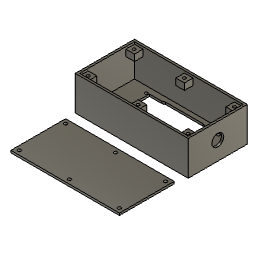
microarcade (Autodesk Fusion 360 design; units mm, degrees)
part number: 2025-05-01-21-42-39-432
Autodesk Fusion 360 part; units mm, degrees
sketch "Sketch1" plane through (0, 0, 0) normal (0, 0, 1) x (1, 0, 0)
  line L0 (33.5, -19.65) -> (-33.5, -19.65) construction
  line L1 (-33.5, -19.65) -> (-33.5, 19.65) construction
  line L2 (-33.5, 19.65) -> (33.5, 19.65) construction
  line L3 (33.5, 19.65) -> (33.5, -19.65) construction
  line L4 (33.5, -19.65) -> (-33.5, 19.65) construction
  line L5 (-33.5, -19.65) -> (33.5, 19.65) construction
  circle A0 centre (-33.5, 19.65) radius 1.375
  circle A1 centre (33.5, 19.65) radius 1.375
  circle A2 centre (-33.5, -19.65) radius 1.375
  circle A3 centre (33.5, -19.65) radius 1.375
  line L6 (31.375, -18.9) -> (-31.375, -18.9) construction
  line L7 (-31.375, -18.9) -> (-31.375, 20.35) construction
  line L8 (-31.375, 20.35) -> (31.375, 20.35) construction
  line L9 (31.375, 20.35) -> (31.375, -18.9)
  line L10 (31.375, -18.9) -> (-31.375, 20.35) construction
  line L11 (-31.375, -18.9) -> (31.375, 20.35) construction
  line L12 (-19.875, 22) -> (-19.875, -25) construction
  line L13 (19.875, 21.8233) -> (19.875, -25.5545) construction
  line L14 (-17.375, 22.5455) -> (-17.375, -22.5266) construction
  line L15 (17.375, 23.3898) -> (17.375, -22.6276) construction
  line L16 (0, 20.35) -> (0, 11.4847) construction
  line L17 (-23.2845, 21.35) -> (29, 21.35) construction
  line L18 (17.375, 21.35) -> (19.875, 20.35)
  line L19 (19.875, 20.35) -> (31.375, 20.35)
  line L20 (31.375, -18.9) -> (-31.375, -18.9)
  line L21 (-31.375, 20.35) -> (-19.875, 20.35)
  line L22 (-19.875, 20.35) -> (-17.375, 21.35)
  line L23 (17.375, 21.35) -> (17.375, 22)
  line L24 (-17.375, 21.35) -> (17.375, 21.35)
  line L25 (31.375, 20.35) -> (31.375, -18.9)
  line L26 (-31.375, 20.35) -> (-31.375, -18.9)
  line L27 (52.5, -27.5) -> (-52.5, -27.5)
  line L28 (-52.5, -27.5) -> (-52.5, 27.5)
  line L29 (-52.5, 27.5) -> (52.5, 27.5)
  line L30 (52.5, 27.5) -> (52.5, -27.5)
  line L31 (52.5, -27.5) -> (-52.5, 27.5) construction
  line L32 (-52.5, -27.5) -> (52.5, 27.5) construction
  circle A4 centre (-42.25, -7.5) radius 3.5
  circle A5 centre (42.25, -7.5) radius 3.5
  line L33 (50.5, 25.5) -> (50.5, -25.5)
  line L34 (50.5, -25.5) -> (-50.5, -25.5)
  line L35 (-50.5, -25.5) -> (-50.5, 25.5)
  line L36 (-50.5, 25.5) -> (50.5, 25.5)
  dimension "d1" = 67
  dimension "d2" = 39.3
  dimension "d3" = 2.75
  dimension "d4" = 2.75
  dimension "d5" = 2.75
  dimension "d6" = 2.75
  dimension "d7" = 62.75
  dimension "d8" = 39.25
  dimension "d9" = 11.5
  dimension "d10" = 11.5
  dimension "d12" = 2.5
  dimension "d13" = 2.5
  dimension "d17" = 0.75
  dimension "d18" = 1
  dimension "d19" = 105
  dimension "d20" = 55
  dimension "d29" = 7
  dimension "d30" = 20
  dimension "d31" = 10.25
  dimension "d32" = 7
  dimension "d33" = 20
  dimension "d34" = 10.25
  dimension "d39" = 2
  constraint horizontal L0
  constraint perpendicular L0 L1
  constraint parallel L0 L2
  constraint parallel L1 L3
  constraint coincident L4 origin
  constraint coincident L5 origin
  constraint coincident L1.end L2.start
  constraint coincident L2.end L3.start
  constraint coincident L0.end L1.start
  constraint coincident L0.start L3.end
  constraint horizontal L6
  constraint perpendicular L6 L7
  constraint parallel L6 L8
  constraint parallel L7 L9
  constraint perpendicular L0 L12
  constraint perpendicular L6 L13
  constraint perpendicular L6 L14
  constraint perpendicular L0 L15
  constraint midpoint L8 L16.start
  constraint perpendicular L2 L16
  constraint coincident origin L16
  constraint parallel L8 L17
  constraint coincident L17 L18.start
  constraint coincident L15 L18.start
  constraint coincident L13 L18.end
  constraint coincident L8 L18.end
  constraint coincident L8 L21.end
  constraint coincident L12 L21.end
  constraint coincident L14 L22.end
  constraint coincident L17 L22.end
  constraint coincident L15 L23.end
  constraint perpendicular L17 L23
  constraint horizontal L27
  constraint perpendicular L27 L28
  constraint parallel L27 L29
  constraint parallel L28 L30
  constraint coincident L31 origin
  constraint coincident L32 origin
  measures "d1" distance of L1.end L2.end
  measures "d2" distance of L0.end L1.end
  measures "d3" diameter of A0
  measures "d4" diameter of A1
  measures "d5" diameter of A2
  measures "d6" diameter of A3
  measures "d7" distance of L7.end L8.end
  measures "d8" distance of L6.end L7.end
  measures "d9" distance of L7 L12
  measures "d10" distance of L9 L13
  measures "d12" distance of L12 L14
  measures "d13" distance of L13 L15
  measures "d17" distance of L0 L6
  measures "d18" distance of L8 L17
  measures "d19" distance of L28.end L29.end
  measures "d20" distance of L27.end L28.end
  measures "d29" diameter of A4
  measures "d30" distance of L27 A4.centre
  measures "d31" distance of L28 A4.centre
  measures "d32" diameter of A5
  measures "d33" distance of L27 A5.centre
  measures "d34" distance of L30 A5.centre
extrude "Extrude1" add sketch "Sketch1" along normal blind 2 contours L27 L28 L29 L30 | A4 | A5 | L33 L34 L35 L36 makes body 1
sketch "Sketch2" plane through (0, 0, 2) normal (0, 0, 1) x (-1, 0, 0)
  circle A0 centre (33.5, 19.65) radius 1.375
  circle A1 centre (33.5, -19.65) radius 1.375
  circle A2 centre (-33.5, -19.65) radius 1.375
  circle A3 centre (-33.5, 19.65) radius 1.375
  line L0 (31.375, -20.35) -> (19.875, -20.35)
  line L1 (19.875, -20.35) -> (17.375, -21.35)
  line L2 (17.375, -21.35) -> (-17.375, -21.35)
  line L3 (-17.375, -21.35) -> (-19.875, -20.35)
  line L4 (-19.875, -20.35) -> (-31.375, -20.35)
  line L5 (-31.375, -20.35) -> (-31.375, 18.9)
  line L6 (-31.375, 18.9) -> (31.375, 18.9)
  line L7 (31.375, 18.9) -> (31.375, -20.35)
  line L8 (-52.5, -27.5) -> (52.5, -27.5)
  line L9 (52.5, -27.5) -> (52.5, 27.5)
  line L10 (52.5, 27.5) -> (-52.5, 27.5)
  line L11 (-52.5, 27.5) -> (-52.5, -27.5)
  line L12 (0, -29) -> (0, 27) construction
  line L13 (22.4113, 21.9) -> (-25, 21.9) construction
  line L14 (9, 7.5969) -> (9, 29.497) construction
  line L15 (-9, 10) -> (-9, 29) construction
  line L16 (11.7573, 19.4) -> (-17.4231, 19.4) construction
  line L17 (9, 19.4) -> (-9, 19.4)
  line L18 (-9, 19.4) -> (-9, 21.9)
  line L19 (-9, 21.9) -> (9, 21.9)
  line L20 (9, 21.9) -> (9, 19.4)
  dimension "d23" = 3
  dimension "d24" = 9
  dimension "d25" = 9
  dimension "d26" = 0.5
  constraint perpendicular L2 L12
  constraint parallel L6 L13
  constraint perpendicular L10 L14
  constraint parallel L12 L15
  constraint horizontal L17
  constraint vertical L18
  constraint horizontal L19
  constraint vertical L20
  constraint coincident L13 L18.end
  constraint coincident L15 L18.end
  constraint coincident L16 L17.start
  constraint coincident L14 L17.start
  measures "d23" distance of L6 L13
  measures "d24" distance of L12 L14
  measures "d25" distance of L12 L15
  measures "d26" distance of L6 L16
extrude "Extrude2" cut sketch "Sketch2" against normal blind 1.75 contours L17 L18 L19 L20 bodies 1
sketch "Sketch3" plane through (0, 0, 0) normal (0, 1, 0) x (1, 0, 0)
extrude "Extrude3" cut sketch "Sketch1" along normal blind 2 contours A5 bodies 1
extrude "Extrude4" cut sketch "Sketch1" along normal blind 2 contours A4 bodies 1
sketch "Sketch4" plane through (0, 0, 0) normal (1, 0, 0) x (0, 1, 0)
sketch "Sketch5" plane through (0, 0, 0) normal (0, 0, 1) x (1, 0, 0)
extrude "Extrude5" add sketch "Sketch1" along normal blind 30 contours L27 L28 L29 L30 bodies 1
sketch "Sketch6" plane through (0, 0, 0) normal (0, 1, 0) x (1, 0, 0)
sketch "Sketch7" plane through (0, 0, 30) normal (0, 0, 1) x (-1, 0, 0)
  line L0 (50.5, 25.5) -> (50.5, -25.5)
  line L1 (50.5, -25.5) -> (-50.5, -25.5)
  line L2 (-50.5, -25.5) -> (-50.5, 25.5)
  line L3 (-50.5, 25.5) -> (50.5, 25.5)
  line L4 (-52.5, -27.5) -> (52.5, -27.5)
  line L5 (52.5, -27.5) -> (52.5, 27.5)
  line L6 (52.5, 27.5) -> (-52.5, 27.5)
  line L7 (-52.5, 27.5) -> (-52.5, -27.5)
  line L8 (-50.5, 25.5) -> (-42.5, 25.5)
  line L9 (-42.5, 25.5) -> (-42.5, 17.5)
  line L10 (-42.5, 17.5) -> (-50.5, 17.5)
  line L11 (-50.5, 17.5) -> (-50.5, 25.5)
  line L12 (50.5, 25.5) -> (42.5, 25.5)
  line L13 (42.5, 25.5) -> (42.5, 17.5)
  line L14 (42.5, 17.5) -> (50.5, 17.5)
  line L15 (50.5, 17.5) -> (50.5, 25.5)
  line L16 (-50.5, -25.5) -> (-42.5, -25.5)
  line L17 (-42.5, -25.5) -> (-42.5, -17.5)
  line L18 (-42.5, -17.5) -> (-50.5, -17.5)
  line L19 (-50.5, -17.5) -> (-50.5, -25.5)
  line L20 (50.5, -25.5) -> (42.5, -25.5)
  line L21 (42.5, -25.5) -> (42.5, -17.5)
  line L22 (42.5, -17.5) -> (50.5, -17.5)
  line L23 (50.5, -17.5) -> (50.5, -25.5)
  line L24 (-4, 25.5) -> (4, 25.5)
  line L25 (4, 25.5) -> (4, 17.5)
  line L26 (4, 17.5) -> (-4, 17.5)
  line L27 (-4, 17.5) -> (-4, 25.5)
  line L28 (0, 40) -> (0, -40) construction
  line L29 (-4, -25.5) -> (4, -25.5)
  line L30 (4, -25.5) -> (4, -17.5)
  line L31 (4, -17.5) -> (-4, -17.5)
  line L32 (-4, -17.5) -> (-4, -25.5)
  line L33 (-46.5, 25.5) -> (-46.5, 17.5) construction
  circle A0 centre (-46.5, 21.5) radius 1.4
  line L34 (0, 25.5) -> (0, 17.5) construction
  circle A1 centre (0, 21.5) radius 1.4
  line L35 (46.5, 25.5) -> (46.5, 17.5) construction
  circle A2 centre (46.5, 21.5) radius 1.4
  line L36 (-46.5, -17.5) -> (-46.5, -25.5) construction
  circle A3 centre (-46.5, -21.5) radius 1.4
  line L37 (0, -17.5) -> (0, -25.5) construction
  circle A4 centre (0, -21.5) radius 1.4
  line L38 (46.5, -17.5) -> (46.5, -25.5) construction
  circle A5 centre (46.5, -21.336) radius 1.4
  dimension "d42" = 8
  dimension "d43" = 8
  dimension "d44" = 8
  dimension "d45" = 8
  dimension "d46" = 8
  dimension "d47" = 8
  dimension "d48" = 8
  dimension "d49" = 8
  dimension "d50" = 8
  dimension "d51" = 8
  dimension "d52" = 4
  dimension "d53" = 8
  dimension "d54" = 8
  dimension "d55" = 4
  dimension "d58" = 2.8
  dimension "d59" = 2.8
  dimension "d60" = 2.8
  dimension "d61" = 2.8
  dimension "d62" = 2.8
  dimension "d63" = 2.8
  constraint horizontal L8
  constraint vertical L9
  constraint horizontal L10
  constraint vertical L11
  constraint coincident L2.end L3.start
  constraint horizontal L12
  constraint vertical L13
  constraint horizontal L14
  constraint vertical L15
  constraint coincident L0.start L3.end
  constraint horizontal L16
  constraint vertical L17
  constraint horizontal L18
  constraint vertical L19
  constraint coincident L1.end L2.start
  constraint horizontal L20
  constraint vertical L21
  constraint horizontal L22
  constraint vertical L23
  constraint coincident L0.end L1.start
  constraint horizontal L24
  constraint vertical L25
  constraint horizontal L26
  constraint vertical L27
  constraint coincident L3 L24.start
  constraint perpendicular L4 L28
  constraint horizontal L29
  constraint vertical L30
  constraint horizontal L31
  constraint vertical L32
  constraint coincident L1 L29.start
  constraint midpoint L8 L33.start
  constraint midpoint L10 L33.end
  constraint midpoint L33 A0.centre
  constraint midpoint L24 L34.start
  constraint midpoint L26 L34.end
  constraint midpoint L34 A1.centre
  constraint midpoint L12 L35.start
  constraint midpoint L14 L35.end
  constraint midpoint L35 A2.centre
  constraint midpoint L18 L36.start
  constraint midpoint L16 L36.end
  constraint midpoint L36 A3.centre
  constraint midpoint L31 L37.start
  constraint midpoint L29 L37.end
  constraint midpoint L37 A4.centre
  constraint midpoint L22 L38.start
  constraint midpoint L20 L38.end
  constraint coincident L38 A5.centre
  measures "d42" distance of L2.end L8.end
  measures "d43" distance of L2.end L10.end
  measures "d44" distance of L0.start L12.end
  measures "d45" distance of L12 L14
  measures "d46" distance of L1.end L16.end
  measures "d47" distance of L1.end L18.end
  measures "d48" distance of L20 L22
  measures "d49" distance of L21 L23
  measures "d50" distance of L24.start L26.end
  measures "d51" distance of L25.end L26.end
  measures "d52" distance of L25 L28
  measures "d53" distance of L29.start L31.end
  measures "d54" distance of L29.start L29.end
  measures "d55" distance of L28 L30
  measures "d58" diameter of A0
  measures "d59" diameter of A1
  measures "d60" diameter of A2
  measures "d61" diameter of A3
  measures "d62" diameter of A4
  measures "d63" diameter of A5
extrude "Extrude6" add sketch "Sketch7" against normal blind 6 contours L0 L3 L12 L13 L14 L15 | L0 L1 L20 L21 L22 L23 | L3 L24 L25 L26 L27 | L2 L3 L8 L9 L10 L11 | L1 L29 L30 L31 L32 | L1 L2 L16 L17 L18 L19 | A0 | A1 | A2 | A3 | A4 | A5 bodies 1
extrude "Extrude7" cut sketch "Sketch7" against normal blind 7 contours A0 | A1 | A2 | A3 | A4 | A5 bodies 1
sketch "Sketch8" plane through (52.5, 0, 0) normal (1, 0, 0) x (0, 1, 0)
  line L0 (-27.5, 0) -> (27.5, 0)
  line L1 (27.5, 0) -> (27.5, 30)
  line L2 (27.5, 30) -> (-27.5, 30)
  line L3 (-27.5, 30) -> (-27.5, 0)
  line L4 (0, 30) -> (0, 0) construction
  circle A0 centre (0, 17) radius 5.5
  dimension "d66" = 11
  dimension "d95" = 13
  constraint midpoint L2 L4.start
  constraint coincident L4.end origin
  measures "d66" diameter of A0
  measures "d95" distance of L4.start A0.centre
extrude "Extrude8" cut sketch "Sketch8" against normal blind 2 contours A0 bodies 1
sketch "Sketch9" plane through (0, 0, 0) normal (0, 0, 1) x (1, 0, 0)
sketch "Sketch11" plane through (0, 0, 0) normal (0, 0, 1) x (1, 0, 0)
  line L0 (-50.5, -38.5133) -> (50.5, -38.5133)
  line L1 (50.5, -38.5133) -> (50.5, -89.5133)
  line L2 (50.5, -89.5133) -> (-50.5, -89.5133)
  line L3 (-50.5, -89.5133) -> (-50.5, -38.5133)
  line L4 (-50.5, -38.5133) -> (-46.5, -38.5133)
  line L5 (-46.5, -38.5133) -> (-46.5, -42.5133) construction
  line L6 (-46.5, -42.5133) -> (-50.5, -42.5133) construction
  line L7 (-50.5, -42.5133) -> (-50.5, -38.5133)
  line L8 (-50.5, -38.5133) -> (0, -38.5133)
  line L9 (0, -89.5133) -> (0, -38.5133) construction
  line L10 (-2, -38.5133) -> (-2, -89.5133) construction
  line L11 (-2, -38.5133) -> (2, -38.5133)
  line L12 (2, -38.5133) -> (2, -42.5133) construction
  line L13 (2, -42.5133) -> (-2, -42.5133) construction
  line L14 (-2, -42.5133) -> (-2, -38.5133) construction
  line L15 (-52.5, 27.5) -> (-52.5, -27.5)
  line L16 (50.5, -38.5133) -> (46.5, -38.5133)
  line L17 (46.5, -38.5133) -> (46.5, -42.5133) construction
  line L18 (46.5, -42.5133) -> (50.5, -42.5133) construction
  line L19 (50.5, -42.5133) -> (50.5, -38.5133)
  line L20 (-50.5, -89.5133) -> (-46.5, -89.5133)
  line L21 (-46.5, -89.5133) -> (-46.5, -85.5133) construction
  line L22 (-46.5, -85.5133) -> (-50.5, -85.5133) construction
  line L23 (-50.5, -85.5133) -> (-50.5, -89.5133)
  line L24 (-2, -89.5133) -> (2, -89.5133)
  line L25 (2, -89.5133) -> (2, -85.5133) construction
  line L26 (2, -85.5133) -> (-2, -85.5133) construction
  line L27 (-2, -85.5133) -> (-2, -89.5133)
  line L28 (50.5, -89.5133) -> (46.5, -89.5133)
  line L29 (46.5, -89.5133) -> (46.5, -85.5133) construction
  line L30 (46.5, -85.5133) -> (50.5, -85.5133) construction
  line L31 (50.5, -85.5133) -> (50.5, -89.5133)
  circle A0 centre (-46.5, -42.5133) radius 1.5
  circle A1 centre (0, -42.5133) radius 1.5
  circle A2 centre (46.5, -42.5133) radius 1.5
  circle A3 centre (-46.5, -85.5133) radius 1.5
  circle A4 centre (0, -85.5133) radius 1.5
  circle A5 centre (46.5, -85.5133) radius 1.5
  line L32 (-50.5, -17.5) -> (-50.5, -25.5)
  dimension "d69" = 51
  dimension "d70" = 101
  dimension "d72" = 4
  dimension "d73" = 4
  dimension "d74" = 2
  dimension "d75" = 4
  dimension "d76" = 4
  dimension "d77" = 4
  dimension "d78" = 4
  dimension "d79" = 4
  dimension "d80" = 4
  dimension "d81" = 4
  dimension "d82" = 4
  dimension "d83" = 4
  dimension "d84" = 4
  dimension "d85" = 3
  dimension "d86" = 3
  dimension "d87" = 3
  dimension "d88" = 3
  dimension "d89" = 3
  dimension "d90" = 3
  constraint horizontal L0
  constraint vertical L1
  constraint horizontal L2
  constraint vertical L3
  constraint horizontal L4
  constraint vertical L5
  constraint horizontal L6
  constraint vertical L7
  constraint midpoint L0 L8.end
  constraint midpoint L2 L9.start
  constraint coincident L0 L10.start
  constraint coincident L2 L10.end
  constraint perpendicular L2 L10
  constraint horizontal L11
  constraint vertical L12
  constraint horizontal L13
  constraint vertical L14
  constraint horizontal L16
  constraint vertical L17
  constraint horizontal L18
  constraint vertical L19
  constraint horizontal L20
  constraint vertical L21
  constraint horizontal L22
  constraint vertical L23
  constraint horizontal L24
  constraint vertical L25
  constraint horizontal L26
  constraint vertical L27
  constraint horizontal L28
  constraint vertical L29
  constraint horizontal L30
  constraint vertical L31
  constraint coincident L5.end L6.start
  constraint midpoint L13 A1.centre
  constraint coincident L17.end L18.start
  constraint coincident L21.end L22.start
  constraint midpoint L26 A4.centre
  constraint coincident L29.end L30.start
  constraint collinear L3 L32
  measures "d69" distance of L0.start L2.end
  measures "d70" distance of L0.start L0.end
  measures "d72" distance of L0.start L6.end
  measures "d73" distance of L0.start L4.end
  measures "d74" distance of L8.end L10.start
  measures "d75" distance of L11.end L12.end
  measures "d76" distance of L12.end L13.end
  measures "d77" distance of L16.end L17.end
  measures "d78" distance of L17.end L18.end
  measures "d79" distance of L2.end L22.end
  measures "d80" distance of L21.end L22.end
  measures "d81" distance of L24.end L25.end
  measures "d82" distance of L25.end L26.end
  measures "d83" distance of L28.end L29.end
  measures "d84" distance of L29.end L30.end
  measures "d85" diameter of A0
  measures "d86" diameter of A1
  measures "d87" diameter of A2
  measures "d88" diameter of A3
  measures "d89" diameter of A4
  measures "d90" diameter of A5
extrude "Extrude9" add sketch "Sketch11" along normal blind 2 separate body makes body 2
extrude "Extrude10" add sketch "Sketch7" along normal blind 2 contours L4 L5 L6 L7 bodies 1
sketch "Sketch12" plane through (0, -27.5, 0) normal (0, -1, 0) x (1, 0, 0)
  line L0 (-52.5, 0) -> (52.5, 0)
  line L1 (52.5, 0) -> (52.5, 32)
  line L2 (52.5, 32) -> (-52.5, 32)
  line L3 (-52.5, 32) -> (-52.5, 0)
sketch "Sketch13" plane through (0, 0, 0) normal (0, 1, 0) x (1, 0, 0)
equation "d4 = d3"
equation "d5 = d3"
equation "d6 = d3"
equation "d10 = d9"
equation "d13 = d12"
equation "d25 = d24"
equation "d31 = d34"
equation "d32 = d29"
equation "d33 = d30"
equation "d42 = d43"
equation "d44 = d42"
equation "d45 = d43"
equation "d46 = d43"
equation "d47 = d43"
equation "d48 = d43"
equation "d49 = d43"
equation "d50 = d43"
equation "d51 = d43"
equation "d52 = d43 / 2"
equation "d53 = d43"
equation "d54 = d43"
equation "d55 = d43 / 2"
equation "d59 = d58"
equation "d60 = d58"
equation "d61 = d58"
equation "d62 = d58"
equation "d63 = d58"
equation "d73 = d72"
equation "d74 = d73 / 2"
equation "d75 = d72"
equation "d76 = d72"
equation "d77 = d72"
equation "d78 = d72"
equation "d79 = d72"
equation "d80 = d72"
equation "d81 = d72"
equation "d82 = d72"
equation "d83 = d72"
equation "d84 = d72"
equation "d86 = d85"
equation "d87 = d85"
equation "d88 = d85"
equation "d89 = d85"
equation "d90 = d85"
